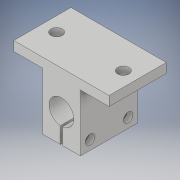
# Autodesk Inventor part: WaterPumpHolder
Saved by Autodesk Inventor 2018 (Build 220112000, 112)
## iProperties
Created: 2016-07-29
Part Number: WaterPumpHolder
Material: Generic
Document SubType Name: Modeling
Designer: reinert
Density: 1 g/cm^3
Appearance: Default
Author: reinert
Autodesk Inventor part; units mm, degrees
ref_plane "YZ Plane" through (0, 0, 0) normal (1, 0, 0) x (0, 1, 0)
ref_plane "XZ Plane" through (0, 0, 0) normal (0, 1, 0) x (-1, 0, 0)
ref_plane "XY Plane" through (0, 0, 0) normal (0, 0, 1) x (1, 0, 0)
sketch "Sketch1" plane through (0, 0, 0) normal (0, 1, 0) x (-1, 0, 0)
  line L0 (5, 0) -> (25, 0)
  arc A0 (15.5, -21.4807) -> (14.5, -21.4807) centre (15, -15) ccw
  line L1 (14.5, -21.4807) -> (14.5, -30)
  line L2 (15.5, -30) -> (15.5, -21.4807)
  line L3 (14.5, -20.3939) -> (15.5, -30) construction
  line L4 (14.5, -30) -> (15.386, -21.4885) construction
  line L5 (25, -30) -> (15.5, -30)
  line L6 (14.5, -30) -> (5, -30)
  line L7 (25, 0) -> (25, -30)
  line L8 (5, 0) -> (5, -30)
  line L9 (25, 0) -> (40, 0)
  line L10 (40, 0) -> (40, 5)
  line L11 (5, 0) -> (-10, 0)
  line L12 (-10, 0) -> (-10, 5)
  line L13 (-10, 5) -> (40, 5)
  point P0 (0, 0)
  point P1 (15, -25.1969)
  dimension "d2" = 13
  dimension "d26" = 15
  dimension "d28" = 15
  constraints: 28 end point, 4 perpendicular, 3 horizontal, 3 parallel, 2 point on circle, 1 centre point, 1 midpoint, 1 point on line
  measures "d2" diameter of A0
  measures "d26" distance of L0.end L9.end
  measures "d28" distance of L0.start L11.end
extrude "Extrusion1" add sketch "Sketch1" along normal blind 30
hole "Hole1" at (-5, 25, -25) direction (-1, 0, 0) diameter 3 end through all counterbore diameter 5 counterbore depth 3
hole "Hole2" at (-5, 5, -25) direction (-1, 0, 0) diameter 3 end through all counterbore diameter 5 counterbore depth 3
sketch "Sketch2" plane through (-25, 0, -30) normal (-1, 0, 0) x (0, 0, 1)
  circle A0 centre (5, 25) radius 1.5 projected
  line L0 (3.9359, 27.9014) -> (6.9806, 27.3722)
  line L1 (6.9806, 27.3722) -> (8.0447, 24.4708)
  line L2 (8.0447, 24.4708) -> (6.0641, 22.0986)
  line L3 (6.0641, 22.0986) -> (3.0194, 22.6278)
  line L4 (3.0194, 22.6278) -> (1.9553, 25.5292)
  line L5 (1.9553, 25.5292) -> (3.9359, 27.9014)
  circle A1 centre (5, 5) radius 1.5 projected
  line L6 (5, 8.0137) -> (7.61, 6.5069)
  line L7 (7.61, 6.5069) -> (7.61, 3.4931)
  line L8 (7.61, 3.4931) -> (5, 1.9863)
  line L9 (5, 1.9863) -> (2.39, 3.4931)
  line L10 (2.39, 3.4931) -> (2.39, 6.5069)
  line L11 (2.39, 6.5069) -> (5, 8.0137)
  point P0 (30, 0)
  constraints: 24 end point, 2 coincident, 26 other
extrude "Extrusion2" cut sketch "Sketch2" against normal blind 3
hole "Hole3" at (-32.5, 15, 0) direction (0, 0, 1) diameter 6 end through all
hole "Hole4" at (2.5, 15, 0) direction (0, 0, 1) diameter 6 end through all
body "Solid1"
